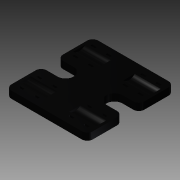
# Autodesk Inventor part: EFFECTOR BEARING PLATE
Saved by Autodesk Inventor 2013 (Build 170138000, 138)
## iProperties
Created: 2014-03-03
Part Number: EFFECTOR BEARING PLATE
Material: Generic
Document SubType Name: Modeling
Designer: employee
Density: 1 g/cm^3
Author: employee
Autodesk Inventor part; units mm, degrees
ref_plane "YZ Plane" through (0, 0, 0) normal (1, 0, 0) x (0, 1, 0)
ref_plane "XZ Plane" through (0, 0, 0) normal (0, 1, 0) x (-1, 0, 0)
ref_plane "XY Plane" through (0, 0, 0) normal (0, 0, 1) x (1, 0, 0)
sketch "Sketch1" plane through (0, 0, 0) normal (0, 0, 1) x (1, 0, 0)
  line L0 (-37.5, 40) -> (37.5, 40)
  line L1 (37.5, 40) -> (37.5, -40)
  line L2 (37.5, -40) -> (-37.5, -40)
  line L3 (-37.5, -40) -> (-37.5, 40)
  point P0 (0, 0)
  point P1 (37.5, 0)
  point P2 (0, 40)
  dimension "d0" = 75
  dimension "d2" = 80
  constraints: 8 end point, 2 midpoint, 2 parallel, 1 horizontal, 1 horizontal alignment, 1 perpendicular, 1 vertical alignment
  measures "d0" distance of L1.end L2.end
  measures "d2" distance of L0.end L1.end
extrude "Extrusion1" add sketch "Sketch1" along normal blind 6.477
sketch "Sketch2" plane through (0, 0, 6.477) normal (0, 0, 1) x (1, 0, 0)
  line L0 (-37.5, 40) -> (-37.5, -40) projected
  line L1 (-11, 19.6967) -> (11, 19.6967) construction
  line L2 (11, 19.6967) -> (11, -19.6967) construction
  line L3 (11, -19.6967) -> (-11, -19.6967) construction
  line L4 (-11, -19.6967) -> (-11, 19.6967) construction
  line L5 (-11, 19.6967) -> (-35, 19.6967)
  line L6 (-35, 19.6967) -> (-35, 30.3033)
  line L7 (-35, 30.3033) -> (-11, 30.3033)
  line L8 (-11, 30.3033) -> (-11, 19.6967)
  line L9 (11, 19.6967) -> (35, 19.6967)
  line L10 (35, 19.6967) -> (35, 30.3033)
  line L11 (35, 30.3033) -> (11, 30.3033)
  line L12 (11, 30.3033) -> (11, 19.6967)
  line L13 (-11, -19.6967) -> (-35, -19.6967)
  line L14 (-35, -19.6967) -> (-35, -30.3033)
  line L15 (-35, -30.3033) -> (-11, -30.3033)
  line L16 (-11, -30.3033) -> (-11, -19.6967)
  line L17 (11, -19.6967) -> (35, -19.6967)
  line L18 (35, -19.6967) -> (35, -30.3033)
  line L19 (35, -30.3033) -> (11, -30.3033)
  line L20 (11, -30.3033) -> (11, -19.6967)
  circle A0 centre (-11, 25) radius 7.5 construction
  line L21 (-11, 25) -> (-5.6967, 19.6967) construction
  point P0 (0, 0)
  point P1 (-11, 0)
  point P2 (0, 19.6967)
  dimension "d11" = 15
  dimension "d5" = 50
  dimension "d7" = 24
  dimension "d9" = 2.5
  dimension "d10" = 45
  constraints: 42 end point, 10 parallel, 6 equal length, 5 horizontal, 5 perpendicular, 3 midpoint, 2 horizontal alignment, 1 coincident, 1 vertical alignment, 3 other
  measures "d5" distance between parallel lines of L7 L13
  measures "d7" distance of L6.end L7.end
  measures "d9" distance between parallel lines of L6 L0
  measures "d10" angle of L21 L8
extrude "Extrusion2" cut sketch "Sketch2" against normal through all
sketch "Sketch3" plane through (-35, 19.6967, 6.477) normal (1, 0, 0) x (0, 0, -1)
  line L0 (6.477, 10.6066) -> (6.477, 0) projected
  line L1 (0, 10.6066) -> (6.477, 10.6066) projected
  line L2 (0, 0) -> (0, 10.6066) projected
  line L3 (0, 0) -> (6.477, 0) projected
  line L4 (6.477, -39.3934) -> (6.477, -50) projected
  line L5 (0, -39.3934) -> (6.477, -39.3934) projected
  line L6 (0, -50) -> (0, -39.3934) projected
  line L7 (0, -50) -> (6.477, -50) projected
  arc A0 (0, 0) -> (0, 10.6066) centre (-5.3033, 5.3033) ccw
  arc A1 (0, -50) -> (0, -39.3934) centre (-5.3033, -44.6967) ccw
  point P0 (6.477, -19.6967)
  dimension "d14" = 15
  constraints: 4 end point, 4 point on circle, 2 centre point, 1 equal radius
  measures "d14" diameter of A0
extrude "Extrusion3" add sketch "Sketch3" along normal up to surface (70 mm away) contours L0 L3 A0 L1 | L4 L7 A1 L5
sketch "Sketch4" plane through (0, 0, 6.477) normal (0, 0, 1) x (1, 0, 0)
  line L0 (-35, 19.6967) -> (-35, 30.3033) projected
  line L1 (-35, 30.3033) -> (-11, 30.3033) projected
  line L2 (-11, 30.3033) -> (-11, 19.6967) projected
  line L3 (-28, 32.5) -> (-18, 32.5) construction
  line L4 (-18, 32.5) -> (-18, 17.5) construction
  line L5 (-18, 17.5) -> (-28, 17.5) construction
  line L6 (-28, 17.5) -> (-28, 32.5) construction
  line L7 (-28, 32.5) -> (-32, 32.5)
  line L8 (-32, 32.5) -> (-32, 34)
  line L9 (-32, 34) -> (-28, 34)
  line L10 (-28, 34) -> (-28, 32.5)
  line L11 (-18, 32.5) -> (-14, 32.5)
  line L12 (-14, 32.5) -> (-14, 34)
  line L13 (-14, 34) -> (-18, 34)
  line L14 (-18, 34) -> (-18, 32.5)
  line L15 (-18, 17.5) -> (-14, 17.5)
  line L16 (-14, 17.5) -> (-14, 16)
  line L17 (-14, 16) -> (-18, 16)
  line L18 (-18, 16) -> (-18, 17.5)
  line L19 (-28, 17.5) -> (-32, 17.5)
  line L20 (-32, 17.5) -> (-32, 16)
  line L21 (-32, 16) -> (-28, 16)
  line L22 (-28, 16) -> (-28, 17.5)
  point P0 (0, 0)
  point P1 (-23, 32.5)
  point P2 (-23, 30.3033)
  point P3 (-18, 25)
  point P4 (-11, 25)
  point P5 (-30, 34)
  dimension "d18" = 5
  dimension "d19" = 15
  dimension "d20" = 4
  dimension "d21" = 1.5
  constraints: 40 end point, 10 parallel, 6 equal length, 5 horizontal, 5 midpoint, 5 perpendicular, 1 horizontal alignment, 1 vertical alignment
  measures "d18" distance from line of point (-30, 34) L0
  measures "d19" distance between parallel lines of L19 L7
  measures "d20" distance of L3.start L7.end
  measures "d21" distance of L9.end L3.start
extrude "Extrusion4" cut sketch "Sketch4" against normal through all
mirror "Mirror1" about plane through (0, 0, 0) normal (1, 0, 0) of "Extrusion4"
mirror "Mirror2" about plane through (0, 0, 0) normal (0, 1, 0) of "Extrusion4", "Mirror1"
fillet "Fillet1" radius 5 4 edges at (-37.5, 40, 3.2385) (-37.5, -40, 3.2385) (37.5, -40, 3.2385) (37.5, 40, 3.2385)
sketch "Sketch6" plane through (0, 0, 6.477) normal (0, 0, 1) x (1, 0, 0)
  line L0 (-37.5, 35) -> (-37.5, -35) projected
  line L1 (37.5, -35) -> (37.5, 35) projected
  line L2 (-11, -19.6967) -> (-11, -30.3033) projected
  line L3 (-37.5, 7.5) -> (-22.5, 7.5)
  arc A0 (-22.5, -7.5) -> (-22.5, 7.5) centre (-22.5, 0) ccw
  line L4 (-22.5, -7.5) -> (-37.5, -7.5)
  line L5 (37.5, -7.5) -> (22.5, -7.5)
  arc A1 (22.5, 7.5) -> (22.5, -7.5) centre (22.5, 0) ccw
  line L6 (22.5, 7.5) -> (37.5, 7.5)
  point P0 (0, 0)
  dimension "d31" = 7.5
  dimension "d33" = 15
  constraints: 8 end point, 4 point on circle, 4 point on line, 4 tangent, 2 centre point, 2 equal length, 2 horizontal alignment, 2 perpendicular, 1 collinear, 1 equal radius
  measures "d31" radius of A0
  measures "d33" distance of L3.start L3.end
extrude "Extrusion6" cut sketch "Sketch6" against normal through all
fillet "Fillet3" radius 5 4 edges at (-37.5, -7.5, 3.2385) (-37.5, 7.5, 3.2385) (37.5, 7.5, 3.2385) (37.5, -7.5, 3.2385)
body "Solid1"
